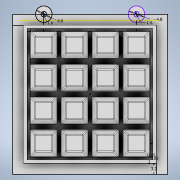
# Autodesk Inventor part: 4x4 keypad flexible cover v2.1
Saved by Autodesk Inventor 2022 (Build 260153000, 153)
## iProperties
Created: 2022-05-03
Part Number: 4x4 keypad flexible cover v2.1
Material: Generic
Document SubType Name: Modeling
Designer: a-dubs
Density: 1 g/cm^3
Appearance: Default
Author: a-dubs
Autodesk Inventor part; units mm, degrees
ref_plane "YZ Plane" through (0, 0, 0) normal (1, 0, 0) x (0, 1, 0)
ref_plane "XZ Plane" through (0, 0, 0) normal (0, 1, 0) x (-1, 0, 0)
ref_plane "XY Plane" through (0, 0, 0) normal (0, 0, 1) x (1, 0, 0)
sketch "Sketch1" plane through (0, 0, 0) normal (0, 1, 0) x (-1, 0, 0)
  line L0 (2.95, 2.95) -> (-2.95, 2.95)
  line L1 (-2.95, 2.95) -> (-2.95, -2.95)
  line L2 (-2.95, -2.95) -> (2.95, -2.95)
  line L3 (2.95, -2.95) -> (2.95, 2.95)
  line L4 (2.95, 2.95) -> (-2.95, -2.95) construction
  line L5 (-2.95, 2.95) -> (2.95, -2.95) construction
  line L6 (-2.95, -2.95) -> (-2.95, -4.75)
  line L7 (-2.95, -4.75) -> (-4.4835, -4.75)
  line L8 (4.4835, 4.75) -> (-4.4835, 4.75)
  line L9 (-4.4835, 4.75) -> (-4.4835, -4.75)
  line L10 (-4.4835, -4.75) -> (4.4835, -4.75)
  line L11 (4.4835, -4.75) -> (4.4835, 4.75)
  line L12 (4.4835, 4.75) -> (-4.4835, -4.75) construction
  line L13 (-4.4835, 4.75) -> (4.4835, -4.75) construction
  circle A0 centre (0, 0) radius 1.7
  line L14 (2.95, 2.95) -> (1.2021, 1.2021)
  circle A1 centre (2.076, 2.076) radius 0.5
  line L15 (0, 0) -> (0, 1)
  circle A2 centre (-2.076, 2.076) radius 0.5
  line L16 (0, 0) -> (-0.5185, 0)
  circle A3 centre (2.076, -2.076) radius 0.5
  circle A4 centre (-2.076, -2.076) radius 0.5
  line L17 (2.95, -2.95) -> (2.95, -2.7)
  line L18 (2.95, -2.7) -> (3.25, -2.7)
  line L19 (3.25, -2.7) -> (3.25, -1.95)
  line L20 (3.25, -1.95) -> (2.95, -1.95)
  line L21 (2.95, -1.95) -> (2.95, -2.7)
  line L22 (-2.95, -2.95) -> (2.95, 2.95) construction
  line L23 (2.95, 2.7) -> (3.25, 2.7)
  line L24 (3.25, 2.7) -> (3.25, 1.95)
  line L25 (3.25, 1.95) -> (2.95, 1.95)
  line L26 (2.95, 1.95) -> (2.95, 2.7)
  line L27 (-2.95, -2.7) -> (-3.25, -2.7)
  line L28 (-3.25, -2.7) -> (-3.25, -1.95)
  line L29 (-3.25, -1.95) -> (-2.95, -1.95)
  line L30 (-3.25, 1.95) -> (-2.95, 1.95)
  line L31 (-2.95, 2.7) -> (-3.25, 2.7)
  line L32 (-3.25, 2.7) -> (-3.25, 1.95)
  line L33 (-2.95, -2.95) -> (-2.95, -3.95)
  line L34 (-2.95, -3.95) -> (-3.95, -3.95)
  line L35 (3.95, 3.95) -> (-3.95, 3.95)
  line L36 (-3.95, 3.95) -> (-3.95, -3.95)
  line L37 (-3.95, -3.95) -> (3.95, -3.95)
  line L38 (3.95, -3.95) -> (3.95, 3.95)
  line L39 (3.95, 3.95) -> (-3.95, -3.95) construction
  line L40 (-3.95, 3.95) -> (3.95, -3.95) construction
  circle A5 centre (0, 0) radius 2.2
  line L41 (2.95, 1.2021) -> (1.2021, 2.95)
  line L42 (-1.2021, 2.95) -> (-2.95, 1.2021)
  line L43 (-2.95, -1.2021) -> (-1.2021, -2.95)
  line L44 (1.2021, -2.95) -> (2.95, -1.2021)
  line L45 (-2.95, 2.95) -> (-3.3036, 3.3036)
  line L46 (3.3036, -3.3036) -> (-3.3036, -3.3036)
  line L47 (-3.3036, -3.3036) -> (-3.3036, 3.3036)
  line L48 (-3.3036, 3.3036) -> (3.3036, 3.3036)
  line L49 (3.3036, 3.3036) -> (3.3036, -3.3036)
  line L50 (3.3036, -3.3036) -> (-3.3036, 3.3036) construction
  line L51 (-3.3036, -3.3036) -> (3.3036, 3.3036) construction
  line L52 (-2.95, 2.95) -> (-3.3036, 2.95)
  point P0 (-1.2021, -2.95)
  dimension "d12" = 3.4
  dimension "d6" = 5.9
  dimension "d7" = 5.9
  dimension "d8" = 1.8
  dimension "d9" = 1.5335
  dimension "d15" = 1
  dimension "d27" = 0.25
  dimension "d28" = 0.3
  dimension "d29" = 0.75
  dimension "d55" = 1
  dimension "d56" = 1
  dimension "d61" = 4.4
  dimension "d64" = 360
  dimension "d72" = 0.5
  constraints: 106 end point, 15 symmetric about line, 10 parallel, 9 midpoint, 9 perpendicular, 7 point on line, 6 horizontal, 5 centre point, 2 coincident, 2 vertical, 19 other
  measures "d6" distance of L0.start L0.end
  measures "d7" distance of L1.end L0.end
  measures "d8" distance of L1.end L6.end
  measures "d9" distance of L6.end L7.end
  measures "d15" diameter of A1
  measures "d27" distance of L2.end L17.end
  measures "d28" distance of L20.end L19.end
  measures "d29" distance of L19.end L18.end
  measures "d55" distance of L1.end L33.end
  measures "d56" distance of L33.end L34.end
  measures "d61" diameter of A5
  measures "d72" distance of L0.end L45.end
extrude "Extrusion8" add sketch "Sketch1" along normal blind 5 contours L34 L36 L35 L38 L37
extrude "Extrusion12" add sketch "Sketch1" along normal blind 1 from surface at 5 contours L14 A1 L41 L0 | L0 L45 L48 L49 L46 L6 L2 L3 L18 L19 L20 L25 L24 L23 | L3 L41 A1 L14 | L41 A1 L3 L44 A3 L2 L43 A4 L1 L42 A2 L0 | L23 L24 L25 L3 | A1 L41 L14 | L14 L41 A1 | L42 A2 L1 L0 | L41 L14 A1 | L41 A1 L14 | L52 L47 L45 | L1 L31 L32 L30 L29 L28 L27 L6 L46 L47 L52 | L42 A2 | A2 L42 | L1 L30 L32 L31 | L3 L2 L44 A3 | L20 L19 L18 L3 | L44 A3 | A3 L44 | L43 A4 L2 L1 | L1 L27 L28 L29 | L43 A4 | A4 L43 | A0 | L34 L36 L35 L38 L37 | A5
chamfer "Chamfer1" distance 0.5 angle 45 4 edges at (0, 5, 3.3036) (-3.3036, 5, 0) (0, 5, -3.3036) (3.3036, 5, 0)
chamfer "Chamfer2" distance 1.5 angle 45 4 edges at (0, 6, 3.95) (3.95, 6, 0) (0, 6, -3.95) (-3.95, 6, 0)
extrude "Extrusion13" add sketch "Sketch1" along normal blind 1 contours L7 L9 L8 L11 L10
fillet "Fillet8" radius 0.5 16 edges at (3.2, 5.25, -3.2) (0, 6, -2.45) (-3.2, 5.25, -3.2) (2.45, 6, 0) (3.2, 5.25, 3.2) (3.95, 4.5, 0) (0, 6, 2.45) (-3.2, 5.25, 3.2) (-2.45, 6, 0) (-3.95, 4.5, 0) (0, 4.5, 3.95) (-3.95, 2.75, 3.95) (-3.95, 2.75, -3.95) (0, 4.5, -3.95) (3.95, 2.75, -3.95) (3.95, 2.75, 3.95)
pattern_linear "Rectangular Pattern2" count 4 spacing 8.967 along (-1, 0, 0) count 4 spacing 9.5 along (0, 0, -1) of "Extrusion13", "Extrusion8", "Chamfer2", "Chamfer1", "Fillet8", "Extrusion12"
chamfer "Chamfer3" [suppressed]
sketch "Sketch3" plane through (0, 1, 0) normal (0, 1, 0) x (1, 0, 0)
  line L0 (4.4835, 33.25) -> (-31.3845, 33.25) projected
  line L1 (-31.3845, 33.25) -> (4.4835, 33.25)
  line L2 (4.4835, 33.25) -> (4.4835, -4.75)
  line L3 (4.4835, -4.75) -> (-31.3845, -4.75)
  line L4 (-31.3845, -4.75) -> (-31.3845, 33.25)
  line L5 (4.4835, -4.75) -> (6.8835, -4.75)
  line L6 (6.8835, -4.75) -> (6.8835, -7.15)
  line L7 (-33.7845, 35.65) -> (6.8835, 35.65)
  line L8 (6.8835, 35.65) -> (6.8835, -7.15)
  line L9 (6.8835, -7.15) -> (-33.7845, -7.15)
  line L10 (-33.7845, -7.15) -> (-33.7845, 35.65)
  line L11 (-33.7845, 35.65) -> (6.8835, -7.15) construction
  line L12 (6.8835, 35.65) -> (-33.7845, -7.15) construction
  point P0 (0, 0)
  point P1 (-13.4505, 14.25)
  dimension "d93" = 2.4
  dimension "d94" = 2.4
  constraints: 24 end point, 4 parallel, 3 horizontal, 3 perpendicular, 2 midpoint
  measures "d93" distance of L2.end L5.end
  measures "d94" distance of L5.end L6.end
extrude "Extrusion14" add sketch "Sketch3" against normal blind 1
sketch "Sketch4" plane through (0, 1, 0) normal (0, 1, 0) x (1, 0, 0)
  line L0 (-3.45, -3.95) -> (3.45, -3.95) projected
  line L1 (3.95, -3.45) -> (3.95, 3.45) projected
  line L2 (3.45, 32.45) -> (-3.45, 32.45) projected
  line L3 (-30.851, 3.45) -> (-30.851, -3.45) projected
  line L4 (-30.851, 32.45) -> (3.95, 32.45)
  line L5 (3.95, 32.45) -> (3.95, -3.95)
  line L6 (3.95, -3.95) -> (-30.851, -3.95)
  line L7 (-30.851, -3.95) -> (-30.851, 32.45)
  line L8 (3.95, -3.95) -> (4.8, -3.95)
  line L9 (4.8, -3.95) -> (4.8, -4.8)
  line L10 (-31.701, 33.3) -> (4.8, 33.3)
  line L11 (4.8, 33.3) -> (4.8, -4.8)
  line L12 (4.8, -4.8) -> (-31.701, -4.8)
  line L13 (-31.701, -4.8) -> (-31.701, 33.3)
  line L14 (-31.701, 33.3) -> (4.8, -4.8) construction
  line L15 (4.8, 33.3) -> (-31.701, -4.8) construction
  line L16 (0, -3.95) -> (0, 0)
  line L17 (-3.45, -3.95) -> (3.45, -3.95) projected
  line L18 (0, 0) -> (4.8, 0)
  line L19 (3.95, 0) -> (0, 0)
  line L20 (-30.851, 32.45) -> (-30.851, 33.3)
  line L21 (-30.851, 32.45) -> (-31.701, 32.45)
  line L22 (4.8, -4.8) -> (4.8, -5.8)
  line L23 (4.8, -5.8) -> (5.8, -5.8)
  line L24 (-31.701, 33.3) -> (-32.701, 33.3)
  line L25 (-32.701, 33.3) -> (-32.701, 34.3)
  line L26 (-32.701, 34.3) -> (5.8, 34.3)
  line L27 (5.8, 34.3) -> (5.8, -5.8)
  line L28 (5.8, -5.8) -> (-32.701, -5.8)
  line L29 (-32.701, -5.8) -> (-32.701, 34.3)
  line L30 (5.8, -5.8) -> (5.8, -9)
  line L31 (5.8, -9) -> (9, -9)
  line L32 (-32.701, 34.3) -> (-35.901, 34.3)
  line L33 (-35.901, 34.3) -> (-35.901, 37.5)
  line L34 (9, -9) -> (-35.901, -9)
  line L35 (-35.901, -9) -> (-35.901, 37.5)
  line L36 (-35.901, 37.5) -> (9, 37.5)
  line L37 (9, 37.5) -> (9, -9)
  line L38 (-22.951, 31.95) -> (-22.951, 32.45)
  line L39 (-22.951, 32.45) -> (-30.851, 32.45)
  line L40 (-3.9503, 31.95) -> (-3.9503, 32.45)
  line L41 (-3.9503, 32.45) -> (3.95, 32.45)
  line L42 (0, 32.45) -> (0, 35.65)
  line L43 (-33.7845, 35.65) -> (6.8835, 35.65) projected
  line L44 (-23.451, 32.45) -> (-30.351, 32.45) projected
  line L45 (-26.901, 32.45) -> (-26.901, 37.5)
  circle A0 centre (-26.901, 37.5) radius 0.8
  circle A1 centre (-26.901, 37.5) radius 2.4
  circle A2 centre (0, 37.5) radius 0.8
  circle A3 centre (0, 37.5) radius 2.4
  point P0 (-30.851, 0)
  point P1 (-13.4505, 14.25)
  point P2 (2.4, 37.5)
  point P3 (-2.4, 37.5)
  point P4 (-0.8, 37.5)
  point P5 (0.8, 37.5)
  point P6 (-24.501, 37.5)
  point P7 (-29.301, 37.5)
  point P8 (-27.701, 37.5)
  point P9 (-26.101, 37.5)
  dimension "d97" = 0.85
  dimension "d98" = 0.85
  dimension "d99" = 1
  dimension "d104" = 3.2
  dimension "d109" = 1.6
  dimension "d110" = 4.8
  dimension "d111" = 1.6
  dimension "d112" = 4.8
  constraints: 78 end point, 18 perpendicular, 12 point on line, 8 equal length, 8 parallel, 7 horizontal, 7 midpoint, 4 centre point, 3 coincident, 3 vertical, 1 collinear
  measures "d97" distance of L5.end L8.end
  measures "d98" distance of L8.end L9.end
  measures "d99" distance of L9.end L22.end
  measures "d104" distance of L23.end L30.end
  measures "d109" diameter of A0
  measures "d110" diameter of A1
  measures "d111" diameter of A2
  measures "d112" diameter of A3
extrude "Extrusion15" add sketch "Sketch4" along normal blind 3.2 contours L11 L10 L42 L26 L27 L23 L22 L9 | L22 L28 L29 L24 L13 L12 | L10 L24 L25 L26 L45 | L10 L45 L26 L42
extrude "Extrusion16" add sketch "Sketch4" against normal blind 1 contours L23 L30 L34 L35 L32 L25 L29 L28 | L27 L26 L42 A3 L36 L37 L31 L30 | L26 L45 A1 L43 A3 L42 | L26 L32 L33 L36 A1 L45 | A3 L43 L42 | L42 L43 A3 | A1 L43 L45 | L45 L43 A1 | L43 A3 L36 A2 | L43 A1 L36 A3 | L45 A0 L36 A1 L43 | L43 A1 L36 A0 L45 | A0 L36 L45 | L45 L36 A0 | L36 A2 picked at (-0.0321, 37.2353)
extrude "Extrusion17" cut sketch "Sketch4" against normal through all contours A0 L36 L45 | L45 L36 A0 | A2 L36 | L36 A2 | L36 A0
extrude "Extrusion18" add sketch "Sketch4" against normal up to surface (1 mm away) contours A3 L36 A2 | A1 L36 A0
body "Solid2"
